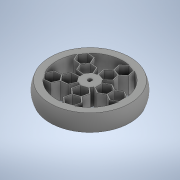
# Autodesk Inventor part: WheelV2
Saved by Autodesk Inventor 2020 (Build 240168000, 168)
## iProperties
Created: 2023-12-12
Part Number: WheelV2
Material: H TPU
Document SubType Name: Modeling
Designer: smz3rm
Density: 0.941117 g/cm^3
Appearance: Generic(1)
Mass: 20.2958 g
Surface Area: 128.27 cm^2
Volume: 15.8561 cm^3
Author: smz3rm
Autodesk Inventor part; units mm, degrees
ref_plane "YZ Plane" through (0, 0, 0) normal (1, 0, 0) x (0, 1, 0)
ref_plane "XZ Plane" through (0, 0, 0) normal (0, 1, 0) x (-1, 0, 0)
ref_plane "XY Plane" through (0, 0, 0) normal (0, 0, 1) x (1, 0, 0)
sketch "Sketch1" plane through (0, 0, 0) normal (0, 1, 0) x (-1, 0, 0)
  circle A0 centre (0, 0) radius 1.5
  line L0 (-1, 1.118) -> (-1, -1.118)
  circle A1 centre (0, 0) radius 30
  circle A2 centre (0, 0) radius 6.5
  circle A3 centre (0, 0) radius 25
  line L1 (42, 0) -> (-42, 0) projected
  line L2 (-10.8681, -4.9216) -> (-15.1303, -2.4608)
  line L3 (-15.1303, -2.4608) -> (-15.1303, 2.4608)
  line L4 (-15.1303, 2.4608) -> (-10.8681, 4.9216)
  line L5 (-10.8681, 4.9216) -> (-6.6059, 2.4608)
  line L6 (-6.6059, 2.4608) -> (-6.6059, -2.4608)
  line L7 (-6.6059, -2.4608) -> (-10.8681, -4.9216)
  line L8 (-5.8059, -2.9227) -> (-5.8059, 2.9227)
  line L9 (-5.8059, 2.9227) -> (-10.8681, 5.8453)
  line L10 (-10.8681, 5.8453) -> (-15.9303, 2.9227)
  line L11 (-15.9303, 2.9227) -> (-15.9303, -2.9227)
  line L12 (-15.9303, -2.9227) -> (-10.8681, -5.8453)
  line L13 (-10.8681, -5.8453) -> (-5.8059, -2.9227)
  line L14 (-20.1925, 4.9216) -> (-15.9303, 2.4608)
  line L15 (-15.9303, 2.4608) -> (-15.9303, -2.4608)
  line L16 (-15.9303, -2.4608) -> (-20.1925, -4.9216)
  line L17 (-20.1925, -4.9216) -> (-24.4547, -2.4608)
  line L18 (-24.4547, -2.4608) -> (-24.4547, 2.4608)
  line L19 (-24.4547, 2.4608) -> (-20.1925, 4.9216)
  line L20 (-20.1925, 5.8453) -> (-15.1303, 2.9227)
  line L21 (-15.1303, 2.9227) -> (-15.1303, -2.9227)
  line L22 (-15.1303, -2.9227) -> (-20.1925, -5.8453)
  line L23 (-20.1925, -5.8453) -> (-25.2547, -2.9227)
  line L24 (-25.2547, -2.9227) -> (-25.2547, 2.9227)
  line L25 (-25.2547, 2.9227) -> (-20.1925, 5.8453)
  line L26 (-15.5303, 2.6917) -> (-10.8681, 5.3834)
  line L27 (-10.8681, 5.3834) -> (-6.2059, 2.6917)
  line L28 (-6.2059, 2.6917) -> (-6.2059, -2.6917)
  line L29 (-6.2059, -2.6917) -> (-10.8681, -5.3834)
  line L30 (-10.8681, -5.3834) -> (-15.5303, -2.6917)
  line L31 (-15.5303, -2.6917) -> (-15.5303, 2.6917)
  line L32 (-15.5303, -2.6917) -> (-15.5303, 2.6917)
  line L33 (-15.5303, 2.6917) -> (-20.1925, 5.3834)
  line L34 (-20.1925, 5.3834) -> (-24.8547, 2.6917)
  line L35 (-24.8547, 2.6917) -> (-24.8547, -2.6917)
  line L36 (-24.8547, -2.6917) -> (-20.1925, -5.3834)
  line L37 (-20.1925, -5.3834) -> (-15.5303, -2.6917)
  line L38 (2.2008, -12.1424) -> (0.9855, -6.4249)
  line L39 (0.9855, -6.4249) -> (-4.5737, -4.6186)
  line L40 (-4.3817, -5.5221) -> (0.299, -7.043)
  line L41 (0.299, -7.043) -> (1.3223, -11.857)
  line L42 (-2.1431, -16.0537) -> (2.2008, -12.1424)
  line L43 (-4.5737, -4.6186) -> (-8.9177, -8.5298)
  line L44 (-8.0391, -8.8153) -> (-4.3817, -5.5221)
  line L45 (-7.0159, -13.6293) -> (-8.0391, -8.8153)
  line L46 (-8.9177, -8.5298) -> (-7.7023, -14.2474)
  line L47 (-7.7023, -14.2474) -> (-2.1431, -16.0537)
  line L48 (-7.4551, -13.4866) -> (-1.8959, -15.2929)
  line L49 (1.3223, -11.857) -> (-2.3352, -15.1502)
  line L50 (-1.8959, -15.2929) -> (-0.6806, -21.0105)
  line L51 (-2.5824, -15.911) -> (-1.5591, -20.725)
  line L52 (-1.5591, -20.725) -> (-5.2166, -24.0182)
  line L53 (-0.6806, -21.0105) -> (-5.0245, -24.9218)
  line L54 (-5.2166, -24.0182) -> (-9.8973, -22.4973)
  line L55 (-5.0245, -24.9218) -> (-10.5837, -23.1155)
  line L56 (-10.5837, -23.1155) -> (-11.7991, -17.3979)
  line L57 (-9.8973, -22.4973) -> (-10.9205, -17.6833)
  line L58 (-10.9205, -17.6833) -> (-7.2631, -14.3902)
  line L59 (-11.7991, -17.3979) -> (-7.4551, -13.4866)
  line L60 (12.2282, -1.6591) -> (6.4149, -1.0481)
  line L61 (6.4149, -1.0481) -> (2.9791, -5.7771)
  line L62 (3.8978, -5.8736) -> (6.7907, -1.892)
  line L63 (6.7907, -1.892) -> (11.6853, -2.4065)
  line L64 (14.6058, -6.9991) -> (12.2282, -1.6591)
  line L65 (2.9791, -5.7771) -> (5.3567, -11.1171)
  line L66 (5.8996, -10.3697) -> (3.8978, -5.8736)
  line L67 (10.7942, -10.8842) -> (5.8996, -10.3697)
  line L68 (5.3567, -11.1171) -> (11.17, -11.7281)
  line L69 (11.17, -11.7281) -> (14.6058, -6.9991)
  line L70 (10.5227, -11.2578) -> (13.9585, -6.5289)
  line L71 (11.6853, -2.4065) -> (13.6871, -6.9025)
  line L72 (13.9585, -6.5289) -> (19.7718, -7.1399)
  line L73 (14.3343, -7.3728) -> (19.2289, -7.8872)
  line L74 (19.2289, -7.8872) -> (21.2307, -12.3833)
  line L75 (19.7718, -7.1399) -> (22.1494, -12.4798)
  line L76 (21.2307, -12.3833) -> (18.3378, -16.3649)
  line L77 (22.1494, -12.4798) -> (18.7136, -17.2088)
  line L78 (18.7136, -17.2088) -> (12.9003, -16.5978)
  line L79 (18.3378, -16.3649) -> (13.4432, -15.8505)
  line L80 (13.4432, -15.8505) -> (11.4414, -11.3544)
  line L81 (12.9003, -16.5978) -> (10.5227, -11.2578)
  line L82 (5.3567, 11.1171) -> (2.9791, 5.7771)
  line L83 (2.9791, 5.7771) -> (6.4149, 1.0481)
  line L84 (6.7907, 1.892) -> (3.8978, 5.8736)
  line L85 (3.8978, 5.8736) -> (5.8996, 10.3697)
  line L86 (11.17, 11.7281) -> (5.3567, 11.1171)
  line L87 (6.4149, 1.0481) -> (12.2282, 1.6591)
  line L88 (11.6853, 2.4065) -> (6.7907, 1.892)
  line L89 (13.6871, 6.9025) -> (11.6853, 2.4065)
  line L90 (12.2282, 1.6591) -> (14.6058, 6.9991)
  line L91 (14.6058, 6.9991) -> (11.17, 11.7281)
  line L92 (13.9585, 6.5289) -> (10.5227, 11.2578)
  line L93 (5.8996, 10.3697) -> (10.7942, 10.8842)
  line L94 (10.5227, 11.2578) -> (12.9003, 16.5978)
  line L95 (11.4414, 11.3544) -> (13.4432, 15.8505)
  line L96 (13.4432, 15.8505) -> (18.3378, 16.3649)
  line L97 (12.9003, 16.5978) -> (18.7136, 17.2088)
  line L98 (18.3378, 16.3649) -> (21.2307, 12.3833)
  line L99 (18.7136, 17.2088) -> (22.1494, 12.4798)
  line L100 (22.1494, 12.4798) -> (19.7718, 7.1399)
  line L101 (21.2307, 12.3833) -> (19.2289, 7.8872)
  line L102 (19.2289, 7.8872) -> (14.3343, 7.3728)
  line L103 (19.7718, 7.1399) -> (13.9585, 6.5289)
  line L104 (-8.9177, 8.5298) -> (-4.5737, 4.6186)
  line L105 (-4.5737, 4.6186) -> (0.9855, 6.4249)
  line L106 (0.299, 7.043) -> (-4.3817, 5.5221)
  line L107 (-4.3817, 5.5221) -> (-8.0391, 8.8153)
  line L108 (-7.7023, 14.2474) -> (-8.9177, 8.5298)
  line L109 (0.9855, 6.4249) -> (2.2008, 12.1424)
  line L110 (1.3223, 11.857) -> (0.299, 7.043)
  line L111 (-2.3352, 15.1502) -> (1.3223, 11.857)
  line L112 (2.2008, 12.1424) -> (-2.1431, 16.0537)
  line L113 (-2.1431, 16.0537) -> (-7.7023, 14.2474)
  line L114 (-1.8959, 15.2929) -> (-7.4551, 13.4866)
  line L115 (-8.0391, 8.8153) -> (-7.0159, 13.6293)
  line L116 (-7.4551, 13.4866) -> (-11.7991, 17.3979)
  line L117 (-7.2631, 14.3902) -> (-10.9205, 17.6833)
  line L118 (-10.9205, 17.6833) -> (-9.8973, 22.4973)
  line L119 (-11.7991, 17.3979) -> (-10.5837, 23.1155)
  line L120 (-9.8973, 22.4973) -> (-5.2166, 24.0182)
  line L121 (-10.5837, 23.1155) -> (-5.0245, 24.9218)
  line L122 (-5.0245, 24.9218) -> (-0.6806, 21.0105)
  line L123 (-5.2166, 24.0182) -> (-1.5591, 20.725)
  line L124 (-1.5591, 20.725) -> (-2.5824, 15.911)
  line L125 (-0.6806, 21.0105) -> (-1.8959, 15.2929)
  point P0 (25, 0)
  point P1 (30, 0)
  point P2 (-30, 0)
  point P3 (-10.8681, 0)
  point P4 (-20.1925, 0)
  point P5 (-6.5, 0)
  point P6 (6.5, 0)
  point P7 (-25, 0)
  point P8 (-24.796, -3.1875)
  point P9 (-15.5303, -3.1536)
  point P10 (-5.8059, 2.9227)
  point P11 (-15.5303, 3.1536)
  point P12 (-24.796, 3.1875)
  point P13 (-15.9303, 2.4608)
  point P14 (-15.9303, -2.4608)
  point P15 (-4.5737, -4.6186)
  point P16 (-7.7984, -13.7956)
  point P17 (-10.6939, -22.5974)
  point P18 (6.4149, 1.0481)
  point P19 (14.4179, 6.5771)
  point P20 (21.9339, 11.996)
  point P21 (18.1868, 17.1534)
  point P22 (10.7106, 11.6798)
  point P23 (2.9791, 5.7771)
  point P24 (0.9855, 6.4249)
  point P25 (-1.7999, 15.7447)
  point P26 (-4.6309, 24.5674)
  point P27 (-10.6939, 22.5974)
  point P28 (-7.7984, 13.7956)
  point P29 (21.9339, -11.996)
  point P30 (14.4179, -6.5771)
  point P31 (6.4149, -1.0481)
  point P32 (-1.325, -6.3635)
  point P33 (-2.3352, -15.1502)
  point P34 (-7.0159, -13.6293)
  point P35 (-2.6684, -5.927)
  point P36 (4.8123, -4.3694)
  point P37 (5.6426, -3.2266)
  point P38 (13.6871, -6.9025)
  point P39 (10.7942, -10.8842)
  point P40 (14.3343, -7.3728)
  point P41 (11.4414, -11.3544)
  point P42 (0.9855, -6.4249)
  point P43 (2.9791, -5.7771)
  point P44 (10.7106, -11.6798)
  point P45 (18.1868, -17.1534)
  point P46 (-4.6309, -24.5674)
  point P47 (-1.7999, -15.7447)
  point P48 (-6.4615, -0.7063)
  point P49 (-6.4615, 0.7063)
  point P50 (5.6426, 3.2266)
  point P51 (4.8123, 4.3694)
  point P52 (10.7942, 10.8842)
  point P53 (13.6871, 6.9025)
  point P54 (11.4414, 11.3544)
  point P55 (14.3343, 7.3728)
  point P56 (-1.325, 6.3635)
  point P57 (-2.6684, 5.927)
  point P58 (-7.0159, 13.6293)
  point P59 (-2.3352, 15.1502)
  point P60 (-7.2631, 14.3902)
  point P61 (-2.5824, 15.911)
  point P62 (-2.5824, -15.911)
  point P63 (-7.2631, -14.3902)
  dimension "d0" = 3
  dimension "d1" = 1
  dimension "d2" = 60
  dimension "d3" = 5
  dimension "d4" = 5
  dimension "d25" = 0.8
  dimension "d26" = 0.8
  dimension "d27" = 0.4
  dimension "d28" = 0.4
  dimension "d37" = 360
  constraints: 250 end point, 4 coincident, 2 centre point, 2 point on circle, 2 point on line, 1 vertical, 283 other
  measures "d0" diameter of A0
  measures "d1" distance from line of point (0, 0) L0
  measures "d2" diameter of A1
  measures "d25" distance between parallel lines of L6 L8
  measures "d26" distance between parallel lines of L19 L25
  measures "d27" distance between parallel lines of L10 L26
  measures "d28" distance between parallel lines of L21 L32
extrude "Extrusion1" add sketch "Sketch1" along normal blind 12.7 contours L1 A2 L61 L39 L8 A0 | A0 L1 L8 A2 L105 L83 | L0 L1 A0 | A0 L1 L0 | L83 A2 | A2 L82 L86 L94 L92 L93 L85 L84 L88 L89 L103 L90 L87 | L60 L64 L72 L70 L71 L63 L62 L66 L67 L81 L68 L65 A2 | A2 L61 | L1 A1 L24 L23 A3 L56 L55 L53 L78 L77 L75 | A3 L100 L99 L97 L122 L121 L119 L25 L24 L1 A1 | L8 A2 L28 L1 | L1 L28 A2 L8 | L100 L103 L90 L91 L102 L101 L98 L96 L95 L86 L94 L97 A3 | A3 L97 L99 L100 | L75 L77 L78 A3 | A3 L78 L81 L68 L69 L80 L79 L76 L74 L73 L64 L72 L75 | L28 A2 L1 | L1 A2 L28 | L13 L12 L22 L30 L29 L28 A2 | A2 L28 L27 L26 L20 L10 L9 | L105 A2 | A2 L104 L108 L116 L114 L115 L107 L106 L110 L111 L125 L112 L109 | L103 L92 L94 L86 L91 L90 | L38 L42 L50 L48 L49 L41 L40 L44 L45 L59 L46 L43 A2 | A2 L39 | L64 L69 L68 L81 L70 L72 | L1 L6 L5 L4 L21 L26 L27 L28 A2 | A2 L28 L29 L30 L21 L2 L7 L6 L1 | L122 L125 L112 L113 L124 L123 L120 L118 L117 L108 L116 L119 A3 | A3 L119 L121 L122 | L53 L55 L56 A3 | A3 L56 L59 L46 L47 L58 L57 L54 L52 L51 L42 L50 L53 | L24 L25 A3 L1 | L1 A3 L23 L24 | L22 L23 A3 L36 L37 L12 | L12 L37 L30 L22 | L20 L26 L33 L10 | L10 L33 L34 A3 L25 L20 | L125 L114 L116 L108 L113 L112 | L42 L47 L46 L59 L48 L50 | L1 L35 A3 | A3 L35 L1 | L3 L21 L30 L31 L1 | L1 L31 L26 L21 L3 | L37 L36 L35 L1 L18 L17 L16 L11 | L11 L1 L31 L37 | L33 L31 L1 L11 | L11 L14 L19 L18 L1 L35 L34 L33 picked at (-1.0704, 0.6676) picked at (-1.0705, -0.6676)
sketch "Sketch2" plane through (0, 0, 0) normal (0, 0, 1) x (1, 0, 0)
  line L0 (30, 12.7) -> (-30, 12.7) projected
  line L1 (30, 0) -> (-30, 0) projected
  line L2 (30, 0) -> (-30, 0) projected
  line L3 (0, -2.54) -> (0, 15.24) projected
  line L4 (24.796, 0) -> (24.796, 12.7) projected
  line L5 (30, 0) -> (30, 12.7) projected
  arc A0 (30, 0) -> (30, 12.7) centre (17.3092, 6.35) ccw
  point P0 (0, 0)
  point P1 (-27.5, 12.7)
  point P2 (31.5, 6.35)
  dimension "d39" = 1.5
  constraints: 3 point on circle, 1 centre point
  measures "d39" distance from line of L5 point (31.5, 6.35)
revolve "Revolution1" add sketch "Sketch2" angle 360 about axis through (0, -10, 0) along (0, 1, 0) contours A0 L5
body "Solid1"
